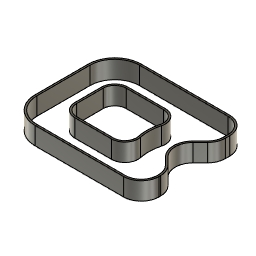
road (Autodesk Fusion 360 design; units mm, degrees)
Autodesk Fusion 360 part; units mm, degrees
sketch "草图1" plane through (0, 0, 0) normal (0, 0, 1) x (1, 0, 0)
  line L0 (0, 30) -> (0, 90)
  line L1 (30, 120) -> (130, 120)
  arc A0 (30, 120) -> (0, 90) centre (30, 90) ccw
  line L2 (30, 0) -> (130, 0)
  line L3 (144.1421, 80.862) -> (135.8579, 72.5777)
  line L4 (135.8579, 44.2934) -> (144.1421, 36.0092)
  line L5 (121.7157, 58.4356) -> (150, 58.4356) construction
  arc A1 (150, 100) -> (130, 120) centre (130, 100) ccw
  line L6 (150, 20) -> (150, 21.867)
  line L7 (150, 95.0041) -> (150, 100)
  arc A2 (144.1421, 80.862) -> (150, 95.0041) centre (130, 95.0041) ccw
  arc A3 (135.8579, 72.5777) -> (135.8579, 44.2934) centre (150, 58.4356) ccw
  arc A4 (150, 21.867) -> (144.1421, 36.0092) centre (130, 21.867) ccw
  arc A5 (130, 0) -> (150, 20) centre (130, 20) ccw
  arc A6 (0, 30) -> (30, 0) centre (30, 30) ccw
  arc A7 (148, 100) -> (130, 118) centre (130, 100) ccw
  line L8 (30, 118) -> (130, 118)
  arc A8 (30, 118) -> (2, 90) centre (30, 90) ccw
  line L9 (2, 30) -> (2, 90)
  arc A9 (2, 30) -> (30, 2) centre (30, 30) ccw
  line L10 (30, 2) -> (130, 2)
  arc A10 (130, 2) -> (148, 20) centre (130, 20) ccw
  line L11 (148, 20) -> (148, 21.867)
  arc A11 (148, 21.867) -> (142.7279, 34.5949) centre (130, 21.867) ccw
  line L12 (134.4437, 42.8792) -> (142.7279, 34.5949)
  arc A12 (134.4437, 73.9919) -> (134.4437, 42.8792) centre (150, 58.4356) ccw
  line L13 (142.7279, 82.2762) -> (134.4437, 73.9919)
  arc A13 (142.7279, 82.2762) -> (148, 95.0041) centre (130, 95.0041) ccw
  line L14 (148, 95.0041) -> (148, 100)
  line L15 (30, 45) -> (30, 75)
  line L16 (45, 90) -> (87.146, 90)
  arc A14 (101.6508, 71.1774) -> (101.0798, 48.1005) centre (150, 58.4356) ccw
  line L17 (45, 30) -> (86.4037, 30)
  arc A15 (45, 90) -> (30, 75) centre (45, 75) ccw
  arc A16 (30, 45) -> (45, 30) centre (45, 45) ccw
  arc A17 (86.4037, 30) -> (101.0798, 48.1005) centre (86.4037, 45) ccw
  arc A18 (101.6508, 71.1774) -> (87.146, 90) centre (87.146, 75) ccw
  line L18 (130, 100) -> (130, 20) construction
  arc A19 (99.7168, 71.6871) -> (87.146, 88) centre (87.146, 75) ccw
  line L19 (45, 88) -> (87.146, 88)
  arc A20 (45, 88) -> (32, 75) centre (45, 75) ccw
  line L20 (32, 45) -> (32, 75)
  arc A21 (32, 45) -> (45, 32) centre (45, 45) ccw
  line L21 (45, 32) -> (86.4037, 32)
  arc A22 (86.4037, 32) -> (99.123, 47.6871) centre (86.4037, 45) ccw
  arc A23 (99.7168, 71.6871) -> (99.123, 47.6871) centre (150, 58.4356) ccw
  point P0 (0, 120)
  point P1 (150, 120)
  point P2 (150, 86.7198)
  point P3 (150, 30.1513)
  point P4 (150, 58.4356)
  dimension "d3" = 120
  dimension "d4" = 150
  dimension "d5" = 30
  dimension "d6" = 90
  dimension "d7" = 40
  dimension "d8" = 40
  dimension "d9" = 20
  dimension "d10" = 20
  dimension "d11" = 20
  dimension "d12" = 20
  dimension "d13" = 30
  dimension "d14" = 2
  dimension "d16" = 15
  dimension "d17" = 15
  dimension "d18" = 20
  dimension "d19" = 41.5644
  dimension "d20" = 2
  constraint vertical L0
  constraint perpendicular L0 L1
  constraint coincident P0 L1
  constraint coincident P0 L0
  constraint tangent L1 A0
  constraint tangent L0 A0
  constraint perpendicular L0 L2
  constraint perpendicular L1 L6
  constraint coincident P2 L6
  constraint perpendicular L5 L6
  constraint coincident L5 P4
  constraint coincident P4 L6
  constraint coincident P1 L1
  constraint coincident P1 L6
  constraint tangent L1 A1
  constraint tangent A1 L6
  constraint collinear L6 L7
  constraint coincident P2 L3
  constraint coincident P2 L7
  constraint tangent L3 A2
  constraint tangent L7 A2
  constraint coincident L5.start L4
  constraint coincident L5.start L3
  constraint tangent L4 A3
  constraint tangent L3 A3
  constraint equal A2 A3
  constraint coincident P3 L4
  constraint coincident P3 L6
  constraint tangent L4 A4
  constraint tangent L6 A4
  constraint tangent L6 A5
  constraint tangent L2 A5
  constraint coincident origin L0
  constraint tangent L2 A6
  constraint tangent L0 A6
  constraint concentric A3 A14
  constraint tangent L16 A15
  constraint tangent L15 A15
  constraint tangent L15 A16
  constraint tangent L17 A16
  constraint equal A15 A16
  constraint tangent L17 A17
  constraint tangent A14 A17
  constraint equal A15 A17
  constraint tangent L16 A18
  constraint tangent A14 A18
  constraint coincident A1.centre A7.centre
  constraint coincident A5.centre A10.centre
  measures "d3" distance of origin P0
  measures "d4" distance of P0 P1
  measures "d5" radius of A0
  measures "d6" angle of L3 L4
  measures "d7" distance of P2 L5.start
  measures "d8" distance of L5.start P3
  measures "d9" radius of A1
  measures "d10" radius of A2
  measures "d11" radius of A4
  measures "d12" radius of A5
  measures "d13" radius of A6
  measures "d16" radius of A15
  measures "d17" radius of A18
  measures "d18" radius of A3
  measures "d19" vertical distance of A1.centre P4
extrude "拉伸1" add sketch "草图1" along normal blind 20 makes body 1 at (63.3333, 120, 6.6667) makes body 2 at (59.0487, 90, 13.3333)
